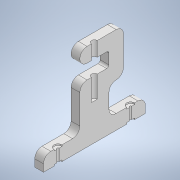
# Autodesk Inventor part: clamp
Saved by Autodesk Inventor 2020 (Build 240168000, 168)
## iProperties
Created: 2020-03-17
Part Number: clamp
Material: Generic
Document SubType Name: Modeling
Designer: erwin
Density: 1 g/cm^3
Appearance: Default
Author: erwin
Autodesk Inventor part; units mm, degrees
ref_plane "YZ Plane" through (0, 0, 0) normal (1, 0, 0) x (0, 1, 0)
ref_plane "XZ Plane" through (0, 0, 0) normal (0, 1, 0) x (-1, 0, 0)
ref_plane "XY Plane" through (0, 0, 0) normal (0, 0, 1) x (1, 0, 0)
sketch "Sketch1" plane through (0, 0, 0) normal (1, 0, 0) x (0, 1, 0)
  line L0 (-10, -70) -> (10, -70)
  line L1 (10, -70) -> (10, 70)
  line L2 (10, 70) -> (-10, 70)
  line L3 (-10, 70) -> (-10, -70)
  line L4 (-10, -70) -> (10, 70) construction
  line L5 (10, -70) -> (-10, 70) construction
  line L6 (10, 0) -> (70, 0)
  line L7 (70, 0) -> (70, 20)
  line L8 (70, 20) -> (10, 20)
  line L9 (10, 20) -> (10, 0)
  line L10 (70, 0) -> (70, -20)
  line L11 (70, -20) -> (10, -20)
  line L12 (10, -20) -> (10, 0)
  line L13 (90, 20) -> (110, 20)
  line L14 (110, 20) -> (110, -20)
  line L15 (110, -20) -> (90, -20)
  line L16 (90, -20) -> (90, 20)
  line L17 (110, -20) -> (50, -20)
  line L18 (50, -20) -> (50, -40)
  line L19 (50, -40) -> (110, -40)
  line L20 (110, -40) -> (110, -20)
  point P0 (0, 0)
  point P1 (90, -20)
  point P2 (70, -20)
  point P3 (50, -20)
  dimension "d0" = 20
  dimension "d1" = 140
  dimension "d2" = 80
  dimension "d3" = 20
  dimension "d17" = 60
  dimension "d18" = 20
  dimension "d19" = 20
  dimension "d20" = 20
  constraints: 42 end point, 8 parallel, 4 horizontal, 4 perpendicular, 3 midpoint, 2 symmetric about line, 1 collinear, 1 point on line
  measures "d0" distance of L2.end L1.end
  measures "d1" distance of L1.end L0.end
  measures "d2" distance between parallel lines of L3 L7
  measures "d3" distance of L6.end L7.end
  measures "d17" distance of L18.end L19.end
  measures "d18" distance of L13.start L13.end
  measures "d19" distance between parallel lines of L7 L16
  measures "d20" distance of L17.end L18.end
extrude "Extrusion1" add sketch "Sketch1" along normal blind 12
fillet "Fillet1" radius 10 10 edges at (6, 10, 70) (6, 10, -70) (6, 10, 20) (6, 10, -20) (6, 70, 20) (6, 90, 20) (6, 110, 20) (6, 110, -40) (6, 50, -40) (6, 50, -20)
fillet "Fillet1" radius 3 2 edges at (6, 70, -20) (6, 90, -20)
sketch "Sketch2" plane through (0, 10, 60) normal (0, 1, 0) x (1, 0, 0)
  line L0 (12, -10) -> (12, 130) projected
  line L1 (0, -10) -> (12, -10) projected
  line L2 (12, 130) -> (0, 130) projected
  point P0 (0, 60)
  point P1 (12, 10)
  point P2 (12, 110)
  dimension "d7" = 100
  dimension "d8" = 20
  dimension "d9" = 20
  constraints: 2 point on line
  measures "d7" distance of point (12, 10) point (12, 110)
  measures "d8" distance from line of L1 point (12, 10)
  measures "d9" distance from line of L2 point (12, 110)
hole "Hole1" at (12, 10, 50) at (12, 10, -50) direction (0, -1, 0) diameter 3 end through all counterbore diameter 11 counterbore depth 2
sketch "Sketch3" plane through (0, 110, 10) normal (0, 1, 0) x (1, 0, 0)
  line L0 (12, -38.5) -> (12, 58.5) projected
  point P0 (0, 10)
  point P1 (12, 10)
  constraints: 1 midpoint
hole "Hole2" at (12, 110, 0) direction (0, -1, 0) diameter 8 depth 70
sketch "Sketch4" plane through (0, -10, -70) normal (0, -1, 0) x (1, 0, 0)
  arc A0 (12, 121.5) -> (12, 118.5) centre (12, 120) ccw projected
  arc A1 (12, 21.5) -> (12, 18.5) centre (12, 20) ccw projected
  point P0 (0, 70)
  constraints: 2 coincident
hole "Hole3" at (12, -10, 50) at (12, -10, -50) direction (0, 1, 0) diameter 11 depth 2
equation "\"d9\" = d8"
body "Solid1"
